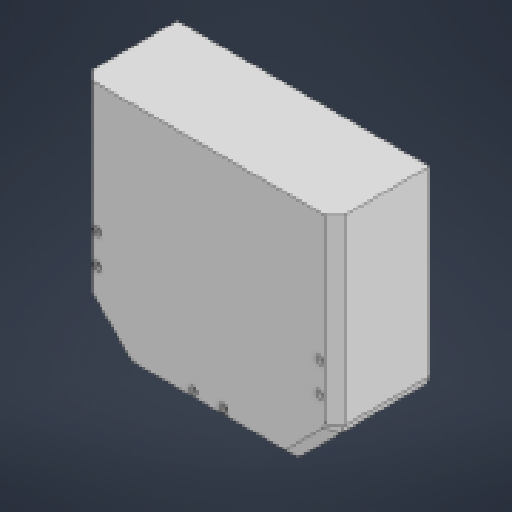
# Autodesk Inventor part: CNC-032-TopCover
Saved by Autodesk Inventor 2026.2 (Build 302298000, 298)
## iProperties
Created: 2026-06-28
Part Number: CNC-032-TopCover
Material: ABS Plastic
Document SubType Name: Modeling
Designer: Kenji
Density: 1.06 g/cm^3
Appearance: Smooth - White
Author: Kenji
Autodesk Inventor part; units mm, degrees
(part 1 of 2)
ref_plane "YZ Plane" through (0, 0, 0) normal (1, 0, 0) x (0, 1, 0)
ref_plane "XZ Plane" through (0, 0, 0) normal (0, 1, 0) x (-1, 0, 0)
ref_plane "XY Plane" through (0, 0, 0) normal (0, 0, 1) x (1, 0, 0)
ref_plane "Work Plane1" through (0, 0, 0) normal (0, 0, 1) x (1, 0, 0)
sketch "Sketch1" plane through (0, 0, 0) normal (0, 0, 1) x (1, 0, 0)
  arc A0 (66.7339, 54.005) -> (67.0931, 54.1538) centre (66.7339, 54.513) ccw construction
  line L0 (66.008, 54.005) -> (66.7339, 54.005) construction
  arc A1 (65.5, 54.513) -> (66.008, 54.005) centre (66.008, 54.513) ccw construction
  line L1 (65.5, 56.862) -> (65.5, 54.513) construction
  arc A2 (65.5, 56.862) -> (64.992, 57.37) centre (64.992, 56.862) ccw construction
  line L2 (64.508, 57.37) -> (64.992, 57.37) construction
  arc A3 (64.508, 57.37) -> (64, 56.862) centre (64.508, 56.862) ccw construction
  line L3 (64, 43.138) -> (64, 56.862) construction
  arc A4 (64, 43.138) -> (64.508, 42.63) centre (64.508, 43.138) ccw construction
  line L4 (64.992, 42.63) -> (64.508, 42.63) construction
  arc A5 (64.992, 42.63) -> (65.5, 43.138) centre (64.992, 43.138) ccw construction
  line L5 (65.5, 45.487) -> (65.5, 43.138) construction
  arc A6 (66.008, 45.995) -> (65.5, 45.487) centre (66.008, 45.487) ccw construction
  line L6 (66.7339, 45.995) -> (66.008, 45.995) construction
  arc A7 (67.0931, 45.8462) -> (66.7339, 45.995) centre (66.7339, 45.487) ccw construction
  line L7 (70.1962, 42.7431) -> (67.0931, 45.8462) construction
  arc A8 (70.345, 42.3839) -> (70.1962, 42.7431) centre (69.837, 42.3839) ccw construction
  line L8 (70.345, 37.6161) -> (70.345, 42.3839) construction
  arc A9 (70.1962, 37.2569) -> (70.345, 37.6161) centre (69.837, 37.6161) ccw construction
  line L9 (67.0931, 34.1538) -> (70.1962, 37.2569) construction
  arc A10 (66.7339, 34.005) -> (67.0931, 34.1538) centre (66.7339, 34.513) ccw construction
  line L10 (66.008, 34.005) -> (66.7339, 34.005) construction
  arc A11 (65.5, 34.513) -> (66.008, 34.005) centre (66.008, 34.513) ccw construction
  line L11 (65.5, 36.862) -> (65.5, 34.513) construction
  arc A12 (65.5, 36.862) -> (64.992, 37.37) centre (64.992, 36.862) ccw construction
  line L12 (64.508, 37.37) -> (64.992, 37.37) construction
  arc A13 (64.508, 37.37) -> (64, 36.862) centre (64.508, 36.862) ccw construction
  line L13 (64, 31.5) -> (64, 36.862) construction
  arc A14 (64, 31.5) -> (65.5, 30) centre (65.5, 31.5) ccw construction
  line L14 (70.862, 30) -> (65.5, 30) construction
  arc A15 (70.862, 30) -> (71.37, 30.508) centre (70.862, 30.508) ccw construction
  line L15 (71.37, 30.992) -> (71.37, 30.508) construction
  arc A16 (71.37, 30.992) -> (70.862, 31.5) centre (70.862, 30.992) ccw construction
  line L16 (68.513, 31.5) -> (70.862, 31.5) construction
  arc A17 (68.005, 32.008) -> (68.513, 31.5) centre (68.513, 32.008) ccw construction
  line L17 (68.005, 32.7339) -> (68.005, 32.008) construction
  arc A18 (68.1538, 33.0931) -> (68.005, 32.7339) centre (68.513, 32.7339) ccw construction
  line L18 (71.2569, 36.1962) -> (68.1538, 33.0931) construction
  arc A19 (71.6161, 36.345) -> (71.2569, 36.1962) centre (71.6161, 35.837) ccw construction
  line L19 (76.3839, 36.345) -> (71.6161, 36.345) construction
  arc A20 (76.7431, 36.1962) -> (76.3839, 36.345) centre (76.3839, 35.837) ccw construction
  line L20 (79.8462, 33.0931) -> (76.7431, 36.1962) construction
  arc A21 (79.995, 32.7339) -> (79.8462, 33.0931) centre (79.487, 32.7339) ccw construction
  line L21 (79.995, 32.008) -> (79.995, 32.7339) construction
  arc A22 (79.487, 31.5) -> (79.995, 32.008) centre (79.487, 32.008) ccw construction
  line L22 (77.138, 31.5) -> (79.487, 31.5) construction
  arc A23 (77.138, 31.5) -> (76.63, 30.992) centre (77.138, 30.992) ccw construction
  line L23 (76.63, 30.508) -> (76.63, 30.992) construction
  arc A24 (76.63, 30.508) -> (77.138, 30) centre (77.138, 30.508) ccw construction
  line L24 (82.5, 30) -> (77.138, 30) construction
  arc A25 (82.5, 30) -> (84, 31.5) centre (82.5, 31.5) ccw construction
  line L25 (84, 36.862) -> (84, 31.5) construction
  arc A26 (84, 36.862) -> (83.492, 37.37) centre (83.492, 36.862) ccw construction
  line L26 (83.008, 37.37) -> (83.492, 37.37) construction
  arc A27 (83.008, 37.37) -> (82.5, 36.862) centre (83.008, 36.862) ccw construction
  line L27 (82.5, 34.513) -> (82.5, 36.862) construction
  arc A28 (81.992, 34.005) -> (82.5, 34.513) centre (81.992, 34.513) ccw construction
  line L28 (81.2661, 34.005) -> (81.992, 34.005) construction
  arc A29 (80.9069, 34.1538) -> (81.2661, 34.005) centre (81.2661, 34.513) ccw construction
  line L29 (77.8038, 37.2569) -> (80.9069, 34.1538) construction
  arc A30 (77.655, 37.6161) -> (77.8038, 37.2569) centre (78.163, 37.6161) ccw construction
  line L30 (77.655, 42.3839) -> (77.655, 37.6161) construction
  arc A31 (77.8038, 42.7431) -> (77.655, 42.3839) centre (78.163, 42.3839) ccw construction
  line L31 (80.9069, 45.8462) -> (77.8038, 42.7431) construction
  arc A32 (81.2661, 45.995) -> (80.9069, 45.8462) centre (81.2661, 45.487) ccw construction
  line L32 (81.992, 45.995) -> (81.2661, 45.995) construction
  arc A33 (82.5, 45.487) -> (81.992, 45.995) centre (81.992, 45.487) ccw construction
  line L33 (82.5, 43.138) -> (82.5, 45.487) construction
  arc A34 (82.5, 43.138) -> (83.008, 42.63) centre (83.008, 43.138) ccw construction
  line L34 (83.492, 42.63) -> (83.008, 42.63) construction
  arc A35 (83.492, 42.63) -> (84, 43.138) centre (83.492, 43.138) ccw construction
  line L35 (84, 56.862) -> (84, 43.138) construction
  arc A36 (84, 56.862) -> (83.492, 57.37) centre (83.492, 56.862) ccw construction
  line L36 (83.008, 57.37) -> (83.492, 57.37) construction
  arc A37 (83.008, 57.37) -> (82.5, 56.862) centre (83.008, 56.862) ccw construction
  line L37 (82.5, 54.513) -> (82.5, 56.862) construction
  arc A38 (81.992, 54.005) -> (82.5, 54.513) centre (81.992, 54.513) ccw construction
  line L38 (81.2661, 54.005) -> (81.992, 54.005) construction
  arc A39 (80.9069, 54.1538) -> (81.2661, 54.005) centre (81.2661, 54.513) ccw construction
  line L39 (77.8038, 57.2569) -> (80.9069, 54.1538) construction
  arc A40 (77.655, 57.6161) -> (77.8038, 57.2569) centre (78.163, 57.6161) ccw construction
  line L40 (77.655, 62.3839) -> (77.655, 57.6161) construction
  arc A41 (77.8038, 62.7431) -> (77.655, 62.3839) centre (78.163, 62.3839) ccw construction
  line L41 (80.9069, 65.8462) -> (77.8038, 62.7431) construction
  arc A42 (81.2661, 65.995) -> (80.9069, 65.8462) centre (81.2661, 65.487) ccw construction
  line L42 (81.992, 65.995) -> (81.2661, 65.995) construction
  arc A43 (82.5, 65.487) -> (81.992, 65.995) centre (81.992, 65.487) ccw construction
  line L43 (82.5, 63.138) -> (82.5, 65.487) construction
  arc A44 (82.5, 63.138) -> (83.008, 62.63) centre (83.008, 63.138) ccw construction
  line L44 (83.492, 62.63) -> (83.008, 62.63) construction
  arc A45 (83.492, 62.63) -> (84, 63.138) centre (83.492, 63.138) ccw construction
  line L45 (84, 68.5) -> (84, 63.138) construction
  arc A46 (84, 68.5) -> (82.5, 70) centre (82.5, 68.5) ccw construction
  line L46 (77.138, 70) -> (82.5, 70) construction
  arc A47 (77.138, 70) -> (76.63, 69.492) centre (77.138, 69.492) ccw construction
  line L47 (76.63, 69.008) -> (76.63, 69.492) construction
  arc A48 (76.63, 69.008) -> (77.138, 68.5) centre (77.138, 69.008) ccw construction
  line L48 (79.487, 68.5) -> (77.138, 68.5) construction
  arc A49 (79.995, 67.992) -> (79.487, 68.5) centre (79.487, 67.992) ccw construction
  line L49 (79.995, 67.2661) -> (79.995, 67.992) construction
  arc A50 (79.8462, 66.9069) -> (79.995, 67.2661) centre (79.487, 67.2661) ccw construction
  line L50 (76.7431, 63.8038) -> (79.8462, 66.9069) construction
  arc A51 (76.3839, 63.655) -> (76.7431, 63.8038) centre (76.3839, 64.163) ccw construction
  line L51 (71.6161, 63.655) -> (76.3839, 63.655) construction
  arc A52 (71.2569, 63.8038) -> (71.6161, 63.655) centre (71.6161, 64.163) ccw construction
  line L52 (68.1538, 66.9069) -> (71.2569, 63.8038) construction
  arc A53 (68.005, 67.2661) -> (68.1538, 66.9069) centre (68.513, 67.2661) ccw construction
  line L53 (68.005, 67.992) -> (68.005, 67.2661) construction
  arc A54 (68.513, 68.5) -> (68.005, 67.992) centre (68.513, 67.992) ccw construction
  line L54 (70.862, 68.5) -> (68.513, 68.5) construction
  arc A55 (70.862, 68.5) -> (71.37, 69.008) centre (70.862, 69.008) ccw construction
  line L55 (71.37, 69.492) -> (71.37, 69.008) construction
  arc A56 (71.37, 69.492) -> (70.862, 70) centre (70.862, 69.492) ccw construction
  line L56 (65.5, 70) -> (70.862, 70) construction
  arc A57 (65.5, 70) -> (64, 68.5) centre (65.5, 68.5) ccw construction
  line L57 (64, 63.138) -> (64, 68.5) construction
  arc A58 (64, 63.138) -> (64.508, 62.63) centre (64.508, 63.138) ccw construction
  line L58 (64.992, 62.63) -> (64.508, 62.63) construction
  arc A59 (64.992, 62.63) -> (65.5, 63.138) centre (64.992, 63.138) ccw construction
  line L59 (65.5, 65.487) -> (65.5, 63.138) construction
  arc A60 (66.008, 65.995) -> (65.5, 65.487) centre (66.008, 65.487) ccw construction
  line L60 (66.7339, 65.995) -> (66.008, 65.995) construction
  arc A61 (67.0931, 65.8462) -> (66.7339, 65.995) centre (66.7339, 65.487) ccw construction
  line L61 (70.1962, 62.7431) -> (67.0931, 65.8462) construction
  arc A62 (70.345, 62.3839) -> (70.1962, 62.7431) centre (69.837, 62.3839) ccw construction
  line L62 (70.345, 57.6161) -> (70.345, 62.3839) construction
  arc A63 (70.1962, 57.2569) -> (70.345, 57.6161) centre (69.837, 57.6161) ccw construction
  line L63 (67.0931, 54.1538) -> (70.1962, 57.2569) construction
  arc A64 (71.6955, 42.1249) -> (72.0649, 40.804) centre (72.252, 41.5684) ccw construction
  line L64 (71.8751, 42.3045) -> (71.6955, 42.1249) construction
  arc A65 (73.196, 41.9351) -> (71.8751, 42.3045) centre (72.4316, 41.748) ccw construction
  arc A66 (74.804, 41.9351) -> (73.196, 41.9351) centre (74, 40) ccw construction
  arc A67 (76.1249, 42.3045) -> (74.804, 41.9351) centre (75.5684, 41.748) ccw construction
  line L65 (76.3045, 42.1249) -> (76.1249, 42.3045) construction
  arc A68 (75.9351, 40.804) -> (76.3045, 42.1249) centre (75.748, 41.5684) ccw construction
  arc A69 (75.9351, 39.196) -> (75.9351, 40.804) centre (74, 40) ccw construction
  arc A70 (76.3045, 37.8751) -> (75.9351, 39.196) centre (75.748, 38.4316) ccw construction
  line L66 (76.1249, 37.6955) -> (76.3045, 37.8751) construction
  arc A71 (74.804, 38.0649) -> (76.1249, 37.6955) centre (75.5684, 38.252) ccw construction
  arc A72 (73.196, 38.0649) -> (74.804, 38.0649) centre (74, 40) ccw construction
  arc A73 (71.8751, 37.6955) -> (73.196, 38.0649) centre (72.4316, 38.252) ccw construction
  line L67 (71.6955, 37.8751) -> (71.8751, 37.6955) construction
  arc A74 (72.0649, 39.196) -> (71.6955, 37.8751) centre (72.252, 38.4316) ccw construction
  arc A75 (72.0649, 40.804) -> (72.0649, 39.196) centre (74, 40) ccw construction
  arc A76 (67.3552, 52.505) -> (67.7144, 52.6538) centre (67.3552, 53.013) ccw construction
  line L68 (71.2569, 56.1962) -> (67.7144, 52.6538) construction
  arc A77 (71.6161, 56.345) -> (71.2569, 56.1962) centre (71.6161, 55.837) ccw construction
  line L69 (76.3839, 56.345) -> (71.6161, 56.345) construction
  arc A78 (76.7431, 56.1962) -> (76.3839, 56.345) centre (76.3839, 55.837) ccw construction
  line L70 (80.2856, 52.6538) -> (76.7431, 56.1962) construction
  arc A79 (80.2856, 52.6538) -> (80.6448, 52.505) centre (80.6448, 53.013) ccw construction
  line L71 (81.992, 52.505) -> (80.6448, 52.505) construction
  arc A80 (82.5, 51.997) -> (81.992, 52.505) centre (81.992, 51.997) ccw construction
  line L72 (82.5, 48.003) -> (82.5, 51.997) construction
  arc A81 (81.992, 47.495) -> (82.5, 48.003) centre (81.992, 48.003) ccw construction
  line L73 (80.6448, 47.495) -> (81.992, 47.495) construction
  arc A82 (80.6448, 47.495) -> (80.2856, 47.3462) centre (80.6448, 46.987) ccw construction
  line L74 (76.7431, 43.8038) -> (80.2856, 47.3462) construction
  arc A83 (76.3839, 43.655) -> (76.7431, 43.8038) centre (76.3839, 44.163) ccw construction
  line L75 (71.6161, 43.655) -> (76.3839, 43.655) construction
  arc A84 (71.2569, 43.8038) -> (71.6161, 43.655) centre (71.6161, 44.163) ccw construction
  line L76 (67.7144, 47.3462) -> (71.2569, 43.8038) construction
  arc A85 (67.7144, 47.3462) -> (67.3552, 47.495) centre (67.3552, 46.987) ccw construction
  line L77 (66.008, 47.495) -> (67.3552, 47.495) construction
  arc A86 (65.5, 48.003) -> (66.008, 47.495) centre (66.008, 48.003) ccw construction
  line L78 (65.5, 51.997) -> (65.5, 48.003) construction
  arc A87 (66.008, 52.505) -> (65.5, 51.997) centre (66.008, 51.997) ccw construction
  line L79 (67.3552, 52.505) -> (66.008, 52.505) construction
  arc A88 (71.6955, 62.1249) -> (72.0649, 60.804) centre (72.252, 61.5684) ccw construction
  line L80 (71.8751, 62.3045) -> (71.6955, 62.1249) construction
  arc A89 (73.196, 61.9351) -> (71.8751, 62.3045) centre (72.4316, 61.748) ccw construction
  arc A90 (74.804, 61.9351) -> (73.196, 61.9351) centre (74, 60) ccw construction
  arc A91 (76.1249, 62.3045) -> (74.804, 61.9351) centre (75.5684, 61.748) ccw construction
  line L81 (76.3045, 62.1249) -> (76.1249, 62.3045) construction
  arc A92 (75.9351, 60.804) -> (76.3045, 62.1249) centre (75.748, 61.5684) ccw construction
  arc A93 (75.9351, 59.196) -> (75.9351, 60.804) centre (74, 60) ccw construction
  arc A94 (76.3045, 57.8751) -> (75.9351, 59.196) centre (75.748, 58.4316) ccw construction
  line L82 (76.1249, 57.6955) -> (76.3045, 57.8751) construction
  arc A95 (74.804, 58.0649) -> (76.1249, 57.6955) centre (75.5684, 58.252) ccw construction
  arc A96 (73.196, 58.0649) -> (74.804, 58.0649) centre (74, 60) ccw construction
  arc A97 (71.8751, 57.6955) -> (73.196, 58.0649) centre (72.4316, 58.252) ccw construction
  line L83 (71.6955, 57.8751) -> (71.8751, 57.6955) construction
  arc A98 (72.0649, 59.196) -> (71.6955, 57.8751) centre (72.252, 58.4316) ccw construction
  arc A99 (72.0649, 60.804) -> (72.0649, 59.196) centre (74, 60) ccw construction
  arc A100 (-66.7339, 45.995) -> (-67.0931, 45.8462) centre (-66.7339, 45.487) ccw construction
  line L84 (-66.008, 45.995) -> (-66.7339, 45.995) construction
  arc A101 (-65.5, 45.487) -> (-66.008, 45.995) centre (-66.008, 45.487) ccw construction
  line L85 (-65.5, 43.138) -> (-65.5, 45.487) construction
  arc A102 (-65.5, 43.138) -> (-64.992, 42.63) centre (-64.992, 43.138) ccw construction
  line L86 (-64.508, 42.63) -> (-64.992, 42.63) construction
  arc A103 (-64.508, 42.63) -> (-64, 43.138) centre (-64.508, 43.138) ccw construction
  line L87 (-64, 56.862) -> (-64, 43.138) construction
  arc A104 (-64, 56.862) -> (-64.508, 57.37) centre (-64.508, 56.862) ccw construction
  line L88 (-64.992, 57.37) -> (-64.508, 57.37) construction
  arc A105 (-64.992, 57.37) -> (-65.5, 56.862) centre (-64.992, 56.862) ccw construction
  line L89 (-65.5, 54.513) -> (-65.5, 56.862) construction
  arc A106 (-66.008, 54.005) -> (-65.5, 54.513) centre (-66.008, 54.513) ccw construction
  line L90 (-66.7339, 54.005) -> (-66.008, 54.005) construction
  arc A107 (-67.0931, 54.1538) -> (-66.7339, 54.005) centre (-66.7339, 54.513) ccw construction
  line L91 (-70.1962, 57.2569) -> (-67.0931, 54.1538) construction
  arc A108 (-70.345, 57.6161) -> (-70.1962, 57.2569) centre (-69.837, 57.6161) ccw construction
  line L92 (-70.345, 62.3839) -> (-70.345, 57.6161) construction
  arc A109 (-70.1962, 62.7431) -> (-70.345, 62.3839) centre (-69.837, 62.3839) ccw construction
  line L93 (-67.0931, 65.8462) -> (-70.1962, 62.7431) construction
  arc A110 (-66.7339, 65.995) -> (-67.0931, 65.8462) centre (-66.7339, 65.487) ccw construction
  line L94 (-66.008, 65.995) -> (-66.7339, 65.995) construction
  arc A111 (-65.5, 65.487) -> (-66.008, 65.995) centre (-66.008, 65.487) ccw construction
  line L95 (-65.5, 63.138) -> (-65.5, 65.487) construction
  arc A112 (-65.5, 63.138) -> (-64.992, 62.63) centre (-64.992, 63.138) ccw construction
  line L96 (-64.508, 62.63) -> (-64.992, 62.63) construction
  arc A113 (-64.508, 62.63) -> (-64, 63.138) centre (-64.508, 63.138) ccw construction
  line L97 (-64, 68.5) -> (-64, 63.138) construction
  arc A114 (-64, 68.5) -> (-65.5, 70) centre (-65.5, 68.5) ccw construction
  line L98 (-70.862, 70) -> (-65.5, 70) construction
  arc A115 (-70.862, 70) -> (-71.37, 69.492) centre (-70.862, 69.492) ccw construction
  line L99 (-71.37, 69.008) -> (-71.37, 69.492) construction
  arc A116 (-71.37, 69.008) -> (-70.862, 68.5) centre (-70.862, 69.008) ccw construction
  line L100 (-68.513, 68.5) -> (-70.862, 68.5) construction
  arc A117 (-68.005, 67.992) -> (-68.513, 68.5) centre (-68.513, 67.992) ccw construction
  line L101 (-68.005, 67.2661) -> (-68.005, 67.992) construction
  arc A118 (-68.1538, 66.9069) -> (-68.005, 67.2661) centre (-68.513, 67.2661) ccw construction
  line L102 (-71.2569, 63.8038) -> (-68.1538, 66.9069) construction
  arc A119 (-71.6161, 63.655) -> (-71.2569, 63.8038) centre (-71.6161, 64.163) ccw construction
  line L103 (-76.3839, 63.655) -> (-71.6161, 63.655) construction
  arc A120 (-76.7431, 63.8038) -> (-76.3839, 63.655) centre (-76.3839, 64.163) ccw construction
  line L104 (-79.8462, 66.9069) -> (-76.7431, 63.8038) construction
  arc A121 (-79.995, 67.2661) -> (-79.8462, 66.9069) centre (-79.487, 67.2661) ccw construction
  line L105 (-79.995, 67.992) -> (-79.995, 67.2661) construction
  arc A122 (-79.487, 68.5) -> (-79.995, 67.992) centre (-79.487, 67.992) ccw construction
  line L106 (-77.138, 68.5) -> (-79.487, 68.5) construction
  arc A123 (-77.138, 68.5) -> (-76.63, 69.008) centre (-77.138, 69.008) ccw construction
  line L107 (-76.63, 69.492) -> (-76.63, 69.008) construction
  arc A124 (-76.63, 69.492) -> (-77.138, 70) centre (-77.138, 69.492) ccw construction
  line L108 (-82.5, 70) -> (-77.138, 70) construction
  arc A125 (-82.5, 70) -> (-84, 68.5) centre (-82.5, 68.5) ccw construction
  line L109 (-84, 63.138) -> (-84, 68.5) construction
  arc A126 (-84, 63.138) -> (-83.492, 62.63) centre (-83.492, 63.138) ccw construction
  line L110 (-83.008, 62.63) -> (-83.492, 62.63) construction
  arc A127 (-83.008, 62.63) -> (-82.5, 63.138) centre (-83.008, 63.138) ccw construction
  line L111 (-82.5, 65.487) -> (-82.5, 63.138) construction
  arc A128 (-81.992, 65.995) -> (-82.5, 65.487) centre (-81.992, 65.487) ccw construction
  line L112 (-81.2661, 65.995) -> (-81.992, 65.995) construction
  arc A129 (-80.9069, 65.8462) -> (-81.2661, 65.995) centre (-81.2661, 65.487) ccw construction
  line L113 (-77.8038, 62.7431) -> (-80.9069, 65.8462) construction
  arc A130 (-77.655, 62.3839) -> (-77.8038, 62.7431) centre (-78.163, 62.3839) ccw construction
  line L114 (-77.655, 57.6161) -> (-77.655, 62.3839) construction
  arc A131 (-77.8038, 57.2569) -> (-77.655, 57.6161) centre (-78.163, 57.6161) ccw construction
  line L115 (-80.9069, 54.1538) -> (-77.8038, 57.2569) construction
  arc A132 (-81.2661, 54.005) -> (-80.9069, 54.1538) centre (-81.2661, 54.513) ccw construction
  line L116 (-81.992, 54.005) -> (-81.2661, 54.005) construction
  arc A133 (-82.5, 54.513) -> (-81.992, 54.005) centre (-81.992, 54.513) ccw construction
  line L117 (-82.5, 56.862) -> (-82.5, 54.513) construction
  arc A134 (-82.5, 56.862) -> (-83.008, 57.37) centre (-83.008, 56.862) ccw construction
  line L118 (-83.492, 57.37) -> (-83.008, 57.37) construction
  arc A135 (-83.492, 57.37) -> (-84, 56.862) centre (-83.492, 56.862) ccw construction
  line L119 (-84, 43.138) -> (-84, 56.862) construction
  arc A136 (-84, 43.138) -> (-83.492, 42.63) centre (-83.492, 43.138) ccw construction
  line L120 (-83.008, 42.63) -> (-83.492, 42.63) construction
  arc A137 (-83.008, 42.63) -> (-82.5, 43.138) centre (-83.008, 43.138) ccw construction
  line L121 (-82.5, 45.487) -> (-82.5, 43.138) construction
  arc A138 (-81.992, 45.995) -> (-82.5, 45.487) centre (-81.992, 45.487) ccw construction
  line L122 (-81.2661, 45.995) -> (-81.992, 45.995) construction
  arc A139 (-80.9069, 45.8462) -> (-81.2661, 45.995) centre (-81.2661, 45.487) ccw construction
  line L123 (-77.8038, 42.7431) -> (-80.9069, 45.8462) construction
  arc A140 (-77.655, 42.3839) -> (-77.8038, 42.7431) centre (-78.163, 42.3839) ccw construction
  line L124 (-77.655, 37.6161) -> (-77.655, 42.3839) construction
  arc A141 (-77.8038, 37.2569) -> (-77.655, 37.6161) centre (-78.163, 37.6161) ccw construction
  line L125 (-80.9069, 34.1538) -> (-77.8038, 37.2569) construction
  arc A142 (-81.2661, 34.005) -> (-80.9069, 34.1538) centre (-81.2661, 34.513) ccw construction
  line L126 (-81.992, 34.005) -> (-81.2661, 34.005) construction
  arc A143 (-82.5, 34.513) -> (-81.992, 34.005) centre (-81.992, 34.513) ccw construction
  line L127 (-82.5, 36.862) -> (-82.5, 34.513) construction
  arc A144 (-82.5, 36.862) -> (-83.008, 37.37) centre (-83.008, 36.862) ccw construction
  line L128 (-83.492, 37.37) -> (-83.008, 37.37) construction
  arc A145 (-83.492, 37.37) -> (-84, 36.862) centre (-83.492, 36.862) ccw construction
  line L129 (-84, 31.5) -> (-84, 36.862) construction
  arc A146 (-84, 31.5) -> (-82.5, 30) centre (-82.5, 31.5) ccw construction
  line L130 (-77.138, 30) -> (-82.5, 30) construction
  arc A147 (-77.138, 30) -> (-76.63, 30.508) centre (-77.138, 30.508) ccw construction
  line L131 (-76.63, 30.992) -> (-76.63, 30.508) construction
  arc A148 (-76.63, 30.992) -> (-77.138, 31.5) centre (-77.138, 30.992) ccw construction
  line L132 (-79.487, 31.5) -> (-77.138, 31.5) construction
  arc A149 (-79.995, 32.008) -> (-79.487, 31.5) centre (-79.487, 32.008) ccw construction
  line L133 (-79.995, 32.7339) -> (-79.995, 32.008) construction
  arc A150 (-79.8462, 33.0931) -> (-79.995, 32.7339) centre (-79.487, 32.7339) ccw construction
  line L134 (-76.7431, 36.1962) -> (-79.8462, 33.0931) construction
  arc A151 (-76.3839, 36.345) -> (-76.7431, 36.1962) centre (-76.3839, 35.837) ccw construction
  line L135 (-71.6161, 36.345) -> (-76.3839, 36.345) construction
  arc A152 (-71.2569, 36.1962) -> (-71.6161, 36.345) centre (-71.6161, 35.837) ccw construction
  line L136 (-68.1538, 33.0931) -> (-71.2569, 36.1962) construction
  arc A153 (-68.005, 32.7339) -> (-68.1538, 33.0931) centre (-68.513, 32.7339) ccw construction
  line L137 (-68.005, 32.008) -> (-68.005, 32.7339) construction
  arc A154 (-68.513, 31.5) -> (-68.005, 32.008) centre (-68.513, 32.008) ccw construction
  line L138 (-70.862, 31.5) -> (-68.513, 31.5) construction
  arc A155 (-70.862, 31.5) -> (-71.37, 30.992) centre (-70.862, 30.992) ccw construction
  line L139 (-71.37, 30.508) -> (-71.37, 30.992) construction
  arc A156 (-71.37, 30.508) -> (-70.862, 30) centre (-70.862, 30.508) ccw construction
  line L140 (-65.5, 30) -> (-70.862, 30) construction
  arc A157 (-65.5, 30) -> (-64, 31.5) centre (-65.5, 31.5) ccw construction
  line L141 (-64, 36.862) -> (-64, 31.5) construction
  arc A158 (-64, 36.862) -> (-64.508, 37.37) centre (-64.508, 36.862) ccw construction
  line L142 (-64.992, 37.37) -> (-64.508, 37.37) construction
  arc A159 (-64.992, 37.37) -> (-65.5, 36.862) centre (-64.992, 36.862) ccw construction
  line L143 (-65.5, 34.513) -> (-65.5, 36.862) construction
  arc A160 (-66.008, 34.005) -> (-65.5, 34.513) centre (-66.008, 34.513) ccw construction
  line L144 (-66.7339, 34.005) -> (-66.008, 34.005) construction
  arc A161 (-67.0931, 34.1538) -> (-66.7339, 34.005) centre (-66.7339, 34.513) ccw construction
  line L145 (-70.1962, 37.2569) -> (-67.0931, 34.1538) construction
  arc A162 (-70.345, 37.6161) -> (-70.1962, 37.2569) centre (-69.837, 37.6161) ccw construction
  line L146 (-70.345, 42.3839) -> (-70.345, 37.6161) construction
  arc A163 (-70.1962, 42.7431) -> (-70.345, 42.3839) centre (-69.837, 42.3839) ccw construction
  line L147 (-67.0931, 45.8462) -> (-70.1962, 42.7431) construction
  arc A164 (-71.6955, 57.8751) -> (-72.0649, 59.196) centre (-72.252, 58.4316) ccw construction
  line L148 (-71.8751, 57.6955) -> (-71.6955, 57.8751) construction
  arc A165 (-73.196, 58.0649) -> (-71.8751, 57.6955) centre (-72.4316, 58.252) ccw construction
  arc A166 (-74.804, 58.0649) -> (-73.196, 58.0649) centre (-74, 60) ccw construction
  arc A167 (-76.1249, 57.6955) -> (-74.804, 58.0649) centre (-75.5684, 58.252) ccw construction
  line L149 (-76.3045, 57.8751) -> (-76.1249, 57.6955) construction
  arc A168 (-75.9351, 59.196) -> (-76.3045, 57.8751) centre (-75.748, 58.4316) ccw construction
  arc A169 (-75.9351, 60.804) -> (-75.9351, 59.196) centre (-74, 60) ccw construction
  arc A170 (-76.3045, 62.1249) -> (-75.9351, 60.804) centre (-75.748, 61.5684) ccw construction
  line L150 (-76.1249, 62.3045) -> (-76.3045, 62.1249) construction
  arc A171 (-74.804, 61.9351) -> (-76.1249, 62.3045) centre (-75.5684, 61.748) ccw construction
  arc A172 (-73.196, 61.9351) -> (-74.804, 61.9351) centre (-74, 60) ccw construction
  arc A173 (-71.8751, 62.3045) -> (-73.196, 61.9351) centre (-72.4316, 61.748) ccw construction
  line L151 (-71.6955, 62.1249) -> (-71.8751, 62.3045) construction
  arc A174 (-72.0649, 60.804) -> (-71.6955, 62.1249) centre (-72.252, 61.5684) ccw construction
  arc A175 (-72.0649, 59.196) -> (-72.0649, 60.804) centre (-74, 60) ccw construction
  arc A176 (-67.3552, 47.495) -> (-67.7144, 47.3462) centre (-67.3552, 46.987) ccw construction
  line L152 (-71.2569, 43.8038) -> (-67.7144, 47.3462) construction
  arc A177 (-71.6161, 43.655) -> (-71.2569, 43.8038) centre (-71.6161, 44.163) ccw construction
  line L153 (-76.3839, 43.655) -> (-71.6161, 43.655) construction
  arc A178 (-76.7431, 43.8038) -> (-76.3839, 43.655) centre (-76.3839, 44.163) ccw construction
  line L154 (-80.2856, 47.3462) -> (-76.7431, 43.8038) construction
  arc A179 (-80.2856, 47.3462) -> (-80.6448, 47.495) centre (-80.6448, 46.987) ccw construction
  line L155 (-81.992, 47.495) -> (-80.6448, 47.495) construction
  arc A180 (-82.5, 48.003) -> (-81.992, 47.495) centre (-81.992, 48.003) ccw construction
  line L156 (-82.5, 51.997) -> (-82.5, 48.003) construction
  arc A181 (-81.992, 52.505) -> (-82.5, 51.997) centre (-81.992, 51.997) ccw construction
  line L157 (-80.6448, 52.505) -> (-81.992, 52.505) construction
  arc A182 (-80.6448, 52.505) -> (-80.2856, 52.6538) centre (-80.6448, 53.013) ccw construction
  line L158 (-76.7431, 56.1962) -> (-80.2856, 52.6538) construction
  arc A183 (-76.3839, 56.345) -> (-76.7431, 56.1962) centre (-76.3839, 55.837) ccw construction
  line L159 (-71.6161, 56.345) -> (-76.3839, 56.345) construction
  arc A184 (-71.2569, 56.1962) -> (-71.6161, 56.345) centre (-71.6161, 55.837) ccw construction
  line L160 (-67.7144, 52.6538) -> (-71.2569, 56.1962) construction
  arc A185 (-67.7144, 52.6538) -> (-67.3552, 52.505) centre (-67.3552, 53.013) ccw construction
  line L161 (-66.008, 52.505) -> (-67.3552, 52.505) construction
  arc A186 (-65.5, 51.997) -> (-66.008, 52.505) centre (-66.008, 51.997) ccw construction
  line L162 (-65.5, 48.003) -> (-65.5, 51.997) construction
  arc A187 (-66.008, 47.495) -> (-65.5, 48.003) centre (-66.008, 48.003) ccw construction
  line L163 (-67.3552, 47.495) -> (-66.008, 47.495) construction
  arc A188 (-71.6955, 37.8751) -> (-72.0649, 39.196) centre (-72.252, 38.4316) ccw construction
  line L164 (-71.8751, 37.6955) -> (-71.6955, 37.8751) construction
  arc A189 (-73.196, 38.0649) -> (-71.8751, 37.6955) centre (-72.4316, 38.252) ccw construction
  arc A190 (-74.804, 38.0649) -> (-73.196, 38.0649) centre (-74, 40) ccw construction
  arc A191 (-76.1249, 37.6955) -> (-74.804, 38.0649) centre (-75.5684, 38.252) ccw construction
  line L165 (-76.3045, 37.8751) -> (-76.1249, 37.6955) construction
  arc A192 (-75.9351, 39.196) -> (-76.3045, 37.8751) centre (-75.748, 38.4316) ccw construction
  arc A193 (-75.9351, 40.804) -> (-75.9351, 39.196) centre (-74, 40) ccw construction
  arc A194 (-76.3045, 42.1249) -> (-75.9351, 40.804) centre (-75.748, 41.5684) ccw construction
  line L166 (-76.1249, 42.3045) -> (-76.3045, 42.1249) construction
  arc A195 (-74.804, 41.9351) -> (-76.1249, 42.3045) centre (-75.5684, 41.748) ccw construction
  arc A196 (-73.196, 41.9351) -> (-74.804, 41.9351) centre (-74, 40) ccw construction
  arc A197 (-71.8751, 42.3045) -> (-73.196, 41.9351) centre (-72.4316, 41.748) ccw construction
  line L167 (-71.6955, 42.1249) -> (-71.8751, 42.3045) construction
  arc A198 (-72.0649, 40.804) -> (-71.6955, 42.1249) centre (-72.252, 41.5684) ccw construction
  arc A199 (-72.0649, 39.196) -> (-72.0649, 40.804) centre (-74, 40) ccw construction
  line L168 (13.138, -10) -> (18.5, -10) construction
  arc A200 (18.5, -10) -> (20, -8.5) centre (18.5, -8.5) ccw construction
  line L169 (20, -8.5) -> (20, -3.138) construction
  arc A201 (20, -3.138) -> (19.492, -2.63) centre (19.492, -3.138) ccw construction
  line L170 (19.492, -2.63) -> (19.008, -2.63) construction
  arc A202 (19.008, -2.63) -> (18.5, -3.138) centre (19.008, -3.138) ccw construction
  line L171 (18.5, -3.138) -> (18.5, -5.487) construction
  arc A203 (17.992, -5.995) -> (18.5, -5.487) centre (17.992, -5.487) ccw construction
  line L172 (17.992, -5.995) -> (17.2661, -5.995) construction
  arc A204 (16.9069, -5.8462) -> (17.2661, -5.995) centre (17.2661, -5.487) ccw construction
  line L173 (16.9069, -5.8462) -> (13.8038, -2.7431) construction
  arc A205 (13.655, -2.3839) -> (13.8038, -2.7431) centre (14.163, -2.3839) ccw construction
  line L174 (13.655, -2.3839) -> (13.655, 2.3839) construction
  arc A206 (13.8038, 2.7431) -> (13.655, 2.3839) centre (14.163, 2.3839) ccw construction
  line L175 (13.8038, 2.7431) -> (16.9069, 5.8462) construction
  arc A207 (17.2661, 5.995) -> (16.9069, 5.8462) centre (17.2661, 5.487) ccw construction
  line L176 (17.2661, 5.995) -> (17.992, 5.995) construction
  arc A208 (18.5, 5.487) -> (17.992, 5.995) centre (17.992, 5.487) ccw construction
  line L177 (18.5, 5.487) -> (18.5, 3.138) construction
  arc A209 (18.5, 3.138) -> (19.008, 2.63) centre (19.008, 3.138) ccw construction
  line L178 (19.008, 2.63) -> (19.492, 2.63) construction
  arc A210 (19.492, 2.63) -> (20, 3.138) centre (19.492, 3.138) ccw construction
  line L179 (20, 3.138) -> (20, 8.5) construction
  arc A211 (20, 8.5) -> (18.5, 10) centre (18.5, 8.5) ccw construction
  line L180 (18.5, 10) -> (13.138, 10) construction
  arc A212 (13.138, 10) -> (12.63, 9.492) centre (13.138, 9.492) ccw construction
  line L181 (12.63, 9.492) -> (12.63, 9.008) construction
  arc A213 (12.63, 9.008) -> (13.138, 8.5) centre (13.138, 9.008) ccw construction
  line L182 (13.138, 8.5) -> (15.487, 8.5) construction
  arc A214 (15.995, 7.992) -> (15.487, 8.5) centre (15.487, 7.992) ccw construction
  line L183 (15.995, 7.992) -> (15.995, 7.2661) construction
  arc A215 (15.8462, 6.9069) -> (15.995, 7.2661) centre (15.487, 7.2661) ccw construction
  line L184 (15.8462, 6.9069) -> (12.7431, 3.8038) construction
  arc A216 (12.3839, 3.655) -> (12.7431, 3.8038) centre (12.3839, 4.163) ccw construction
  line L185 (12.3839, 3.655) -> (7.6161, 3.655) construction
  arc A217 (7.2569, 3.8038) -> (7.6161, 3.655) centre (7.6161, 4.163) ccw construction
  line L186 (7.2569, 3.8038) -> (4.1538, 6.9069) construction
  arc A218 (4.005, 7.2661) -> (4.1538, 6.9069) centre (4.513, 7.2661) ccw construction
  line L187 (4.005, 7.2661) -> (4.005, 7.992) construction
  arc A219 (4.513, 8.5) -> (4.005, 7.992) centre (4.513, 7.992) ccw construction
  line L188 (4.513, 8.5) -> (6.862, 8.5) construction
  arc A220 (6.862, 8.5) -> (7.37, 9.008) centre (6.862, 9.008) ccw construction
  line L189 (7.37, 9.008) -> (7.37, 9.492) construction
  arc A221 (7.37, 9.492) -> (6.862, 10) centre (6.862, 9.492) ccw construction
  line L190 (6.862, 10) -> (-6.862, 10) construction
  arc A222 (-6.862, 10) -> (-7.37, 9.492) centre (-6.862, 9.492) ccw construction
  line L191 (-7.37, 9.492) -> (-7.37, 9.008) construction
  arc A223 (-7.37, 9.008) -> (-6.862, 8.5) centre (-6.862, 9.008) ccw construction
  line L192 (-6.862, 8.5) -> (-4.513, 8.5) construction
  arc A224 (-4.005, 7.992) -> (-4.513, 8.5) centre (-4.513, 7.992) ccw construction
  line L193 (-4.005, 7.992) -> (-4.005, 7.2661) construction
  arc A225 (-4.1538, 6.9069) -> (-4.005, 7.2661) centre (-4.513, 7.2661) ccw construction
  line L194 (-4.1538, 6.9069) -> (-7.2569, 3.8038) construction
  arc A226 (-7.6161, 3.655) -> (-7.2569, 3.8038) centre (-7.6161, 4.163) ccw construction
  line L195 (-7.6161, 3.655) -> (-12.3839, 3.655) construction
  arc A227 (-12.7431, 3.8038) -> (-12.3839, 3.655) centre (-12.3839, 4.163) ccw construction
  line L196 (-12.7431, 3.8038) -> (-15.8462, 6.9069) construction
  arc A228 (-15.995, 7.2661) -> (-15.8462, 6.9069) centre (-15.487, 7.2661) ccw construction
  line L197 (-15.995, 7.2661) -> (-15.995, 7.992) construction
  arc A229 (-15.487, 8.5) -> (-15.995, 7.992) centre (-15.487, 7.992) ccw construction
  line L198 (-15.487, 8.5) -> (-13.138, 8.5) construction
  arc A230 (-13.138, 8.5) -> (-12.63, 9.008) centre (-13.138, 9.008) ccw construction
  line L199 (-12.63, 9.008) -> (-12.63, 9.492) construction
  arc A231 (-12.63, 9.492) -> (-13.138, 10) centre (-13.138, 9.492) ccw construction
  line L200 (-13.138, 10) -> (-18.5, 10) construction
  arc A232 (-18.5, 10) -> (-20, 8.5) centre (-18.5, 8.5) ccw construction
  line L201 (-20, 8.5) -> (-20, 3.138) construction
  arc A233 (-20, 3.138) -> (-19.492, 2.63) centre (-19.492, 3.138) ccw construction
  line L202 (-19.492, 2.63) -> (-19.008, 2.63) construction
  arc A234 (-19.008, 2.63) -> (-18.5, 3.138) centre (-19.008, 3.138) ccw construction
  line L203 (-18.5, 3.138) -> (-18.5, 5.487) construction
  arc A235 (-17.992, 5.995) -> (-18.5, 5.487) centre (-17.992, 5.487) ccw construction
  line L204 (-17.992, 5.995) -> (-17.2661, 5.995) construction
  arc A236 (-16.9069, 5.8462) -> (-17.2661, 5.995) centre (-17.2661, 5.487) ccw construction
  line L205 (-16.9069, 5.8462) -> (-13.8038, 2.7431) construction
  arc A237 (-13.655, 2.3839) -> (-13.8038, 2.7431) centre (-14.163, 2.3839) ccw construction
  line L206 (-13.655, 2.3839) -> (-13.655, -2.3839) construction
  arc A238 (-13.8038, -2.7431) -> (-13.655, -2.3839) centre (-14.163, -2.3839) ccw construction
  line L207 (-13.8038, -2.7431) -> (-16.9069, -5.8462) construction
  arc A239 (-17.2661, -5.995) -> (-16.9069, -5.8462) centre (-17.2661, -5.487) ccw construction
  line L208 (-17.2661, -5.995) -> (-17.992, -5.995) construction
  arc A240 (-18.5, -5.487) -> (-17.992, -5.995) centre (-17.992, -5.487) ccw construction
  line L209 (-18.5, -5.487) -> (-18.5, -3.138) construction
  arc A241 (-18.5, -3.138) -> (-19.008, -2.63) centre (-19.008, -3.138) ccw construction
  line L210 (-19.008, -2.63) -> (-19.492, -2.63) construction
  arc A242 (-19.492, -2.63) -> (-20, -3.138) centre (-19.492, -3.138) ccw construction
  line L211 (-20, -3.138) -> (-20, -8.5) construction
  arc A243 (-20, -8.5) -> (-18.5, -10) centre (-18.5, -8.5) ccw construction
  line L212 (-18.5, -10) -> (-13.138, -10) construction
  arc A244 (-13.138, -10) -> (-12.63, -9.492) centre (-13.138, -9.492) ccw construction
  line L213 (-12.63, -9.492) -> (-12.63, -9.008) construction
  arc A245 (-12.63, -9.008) -> (-13.138, -8.5) centre (-13.138, -9.008) ccw construction
  line L214 (-13.138, -8.5) -> (-15.487, -8.5) construction
  arc A246 (-15.995, -7.992) -> (-15.487, -8.5) centre (-15.487, -7.992) ccw construction
  line L215 (-15.995, -7.992) -> (-15.995, -7.2661) construction
  arc A247 (-15.8462, -6.9069) -> (-15.995, -7.2661) centre (-15.487, -7.2661) ccw construction
  line L216 (-15.8462, -6.9069) -> (-12.7431, -3.8038) construction
  arc A248 (-12.3839, -3.655) -> (-12.7431, -3.8038) centre (-12.3839, -4.163) ccw construction
  line L217 (-12.3839, -3.655) -> (-7.6161, -3.655) construction
  arc A249 (-7.2569, -3.8038) -> (-7.6161, -3.655) centre (-7.6161, -4.163) ccw construction
  line L218 (-7.2569, -3.8038) -> (-4.1538, -6.9069) construction
  arc A250 (-4.005, -7.2661) -> (-4.1538, -6.9069) centre (-4.513, -7.2661) ccw construction
  line L219 (-4.005, -7.2661) -> (-4.005, -7.992) construction
  arc A251 (-4.513, -8.5) -> (-4.005, -7.992) centre (-4.513, -7.992) ccw construction
  line L220 (-4.513, -8.5) -> (-6.862, -8.5) construction
  arc A252 (-6.862, -8.5) -> (-7.37, -9.008) centre (-6.862, -9.008) ccw construction
  line L221 (-7.37, -9.008) -> (-7.37, -9.492) construction
  arc A253 (-7.37, -9.492) -> (-6.862, -10) centre (-6.862, -9.492) ccw construction
  line L222 (-6.862, -10) -> (6.862, -10) construction
  arc A254 (6.862, -10) -> (7.37, -9.492) centre (6.862, -9.492) ccw construction
  line L223 (7.37, -9.492) -> (7.37, -9.008) construction
  arc A255 (7.37, -9.008) -> (6.862, -8.5) centre (6.862, -9.008) ccw construction
  line L224 (6.862, -8.5) -> (4.513, -8.5) construction
  arc A256 (4.005, -7.992) -> (4.513, -8.5) centre (4.513, -7.992) ccw construction
  line L225 (4.005, -7.992) -> (4.005, -7.2661) construction
  arc A257 (4.1538, -6.9069) -> (4.005, -7.2661) centre (4.513, -7.2661) ccw construction
  line L226 (4.1538, -6.9069) -> (7.2569, -3.8038) construction
  arc A258 (7.6161, -3.655) -> (7.2569, -3.8038) centre (7.6161, -4.163) ccw construction
  line L227 (7.6161, -3.655) -> (12.3839, -3.655) construction
  arc A259 (12.7431, -3.8038) -> (12.3839, -3.655) centre (12.3839, -4.163) ccw construction
  line L228 (12.7431, -3.8038) -> (15.8462, -6.9069) construction
  arc A260 (15.995, -7.2661) -> (15.8462, -6.9069) centre (15.487, -7.2661) ccw construction
  line L229 (15.995, -7.2661) -> (15.995, -7.992) construction
  arc A261 (15.487, -8.5) -> (15.995, -7.992) centre (15.487, -7.992) ccw construction
  line L230 (15.487, -8.5) -> (13.138, -8.5) construction
  arc A262 (13.138, -8.5) -> (12.63, -9.008) centre (13.138, -9.008) ccw construction
  line L231 (12.63, -9.008) -> (12.63, -9.492) construction
  arc A263 (12.63, -9.492) -> (13.138, -10) centre (13.138, -9.492) ccw construction
  line L232 (12.3045, -2.1249) -> (12.1249, -2.3045) construction
  arc A264 (10.804, -1.9351) -> (12.1249, -2.3045) centre (11.5684, -1.748) ccw construction
  arc A265 (9.196, -1.9351) -> (10.804, -1.9351) centre (10, 0) ccw construction
  arc A266 (7.8751, -2.3045) -> (9.196, -1.9351) centre (8.4316, -1.748) ccw construction
  line L233 (7.8751, -2.3045) -> (7.6955, -2.1249) construction
  arc A267 (8.0649, -0.804) -> (7.6955, -2.1249) centre (8.252, -1.5684) ccw construction
  arc A268 (8.0649, 0.804) -> (8.0649, -0.804) centre (10, 0) ccw construction
  arc A269 (7.6955, 2.1249) -> (8.0649, 0.804) centre (8.252, 1.5684) ccw construction
  line L234 (7.6955, 2.1249) -> (7.8751, 2.3045) construction
  arc A270 (9.196, 1.9351) -> (7.8751, 2.3045) centre (8.4316, 1.748) ccw construction
  arc A271 (10.804, 1.9351) -> (9.196, 1.9351) centre (10, 0) ccw construction
  arc A272 (12.1249, 2.3045) -> (10.804, 1.9351) centre (11.5684, 1.748) ccw construction
  line L235 (12.1249, 2.3045) -> (12.3045, 2.1249) construction
  arc A273 (11.9351, 0.804) -> (12.3045, 2.1249) centre (11.748, 1.5684) ccw construction
  arc A274 (11.9351, -0.804) -> (11.9351, 0.804) centre (10, 0) ccw construction
  arc A275 (12.3045, -2.1249) -> (11.9351, -0.804) centre (11.748, -1.5684) ccw construction
  line L236 (-12.3045, 2.1249) -> (-12.1249, 2.3045) construction
  arc A276 (-10.804, 1.9351) -> (-12.1249, 2.3045) centre (-11.5684, 1.748) ccw construction
  arc A277 (-9.196, 1.9351) -> (-10.804, 1.9351) centre (-10, 0) ccw construction
  arc A278 (-7.8751, 2.3045) -> (-9.196, 1.9351) centre (-8.4316, 1.748) ccw construction
  line L237 (-7.8751, 2.3045) -> (-7.6955, 2.1249) construction
  arc A279 (-8.0649, 0.804) -> (-7.6955, 2.1249) centre (-8.252, 1.5684) ccw construction
  arc A280 (-8.0649, -0.804) -> (-8.0649, 0.804) centre (-10, 0) ccw construction
  arc A281 (-7.6955, -2.1249) -> (-8.0649, -0.804) centre (-8.252, -1.5684) ccw construction
  line L238 (-7.6955, -2.1249) -> (-7.8751, -2.3045) construction
  arc A282 (-9.196, -1.9351) -> (-7.8751, -2.3045) centre (-8.4316, -1.748) ccw construction
  arc A283 (-10.804, -1.9351) -> (-9.196, -1.9351) centre (-10, 0) ccw construction
  arc A284 (-12.1249, -2.3045) -> (-10.804, -1.9351) centre (-11.5684, -1.748) ccw construction
  line L239 (-12.1249, -2.3045) -> (-12.3045, -2.1249) construction
  arc A285 (-11.9351, -0.804) -> (-12.3045, -2.1249) centre (-11.748, -1.5684) ccw construction
  arc A286 (-11.9351, 0.804) -> (-11.9351, -0.804) centre (-10, 0) ccw construction
  arc A287 (-12.3045, 2.1249) -> (-11.9351, 0.804) centre (-11.748, 1.5684) ccw construction
  arc A288 (2.505, 6.6448) -> (2.6538, 6.2856) centre (3.013, 6.6448) ccw construction
  line L240 (2.6538, 6.2856) -> (6.1962, 2.7431) construction
  arc A289 (6.345, 2.3839) -> (6.1962, 2.7431) centre (5.837, 2.3839) ccw construction
  line L241 (6.345, 2.3839) -> (6.345, -2.3839) construction
  arc A290 (6.1962, -2.7431) -> (6.345, -2.3839) centre (5.837, -2.3839) ccw construction
  line L242 (6.1962, -2.7431) -> (2.6538, -6.2856) construction
  arc A291 (2.6538, -6.2856) -> (2.505, -6.6448) centre (3.013, -6.6448) ccw construction
  line L243 (2.505, -6.6448) -> (2.505, -7.992) construction
  arc A292 (1.997, -8.5) -> (2.505, -7.992) centre (1.997, -7.992) ccw construction
  line L244 (1.997, -8.5) -> (-1.997, -8.5) construction
  arc A293 (-2.505, -7.992) -> (-1.997, -8.5) centre (-1.997, -7.992) ccw construction
  line L245 (-2.505, -7.992) -> (-2.505, -6.6448) construction
  arc A294 (-2.505, -6.6448) -> (-2.6538, -6.2856) centre (-3.013, -6.6448) ccw construction
  line L246 (-2.6538, -6.2856) -> (-6.1962, -2.7431) construction
  arc A295 (-6.345, -2.3839) -> (-6.1962, -2.7431) centre (-5.837, -2.3839) ccw construction
  line L247 (-6.345, -2.3839) -> (-6.345, 2.3839) construction
  arc A296 (-6.1962, 2.7431) -> (-6.345, 2.3839) centre (-5.837, 2.3839) ccw construction
  line L248 (-6.1962, 2.7431) -> (-2.6538, 6.2856) construction
  arc A297 (-2.6538, 6.2856) -> (-2.505, 6.6448) centre (-3.013, 6.6448) ccw construction
  line L249 (-2.505, 6.6448) -> (-2.505, 7.992) construction
  arc A298 (-1.997, 8.5) -> (-2.505, 7.992) centre (-1.997, 7.992) ccw construction
  line L250 (-1.997, 8.5) -> (1.997, 8.5) construction
  arc A299 (2.505, 7.992) -> (1.997, 8.5) centre (1.997, 7.992) ccw construction
  line L251 (2.505, 7.992) -> (2.505, 6.6448) construction
  line L252 (78, 145) -> (-78, 145) construction
  line L253 (0, -10) -> (50.35, -10)
  line L254 (20, 30) -> (84, 30) construction
  line L255 (20, -10) -> (20, 30) construction
  line L256 (50.35, -10) -> (20, -10) projected
  line L257 (50.35, -10) -> (55.7701, -7.7549) projected
  line L258 (81.7549, 18.2299) -> (55.7701, -7.7549) projected
  line L259 (81.7549, 18.2299) -> (84, 23.65) projected
  line L260 (84, 30) -> (84, 23.65) projected
  line L261 (79.2375, 25.2375) -> (40, 25.2375) construction
  line L262 (79.2375, 22.4477) -> (79.2375, 25.2375) construction
  line L263 (51.5523, -5.2375) -> (79.2375, 22.4477) construction
  line L264 (24.7625, -5.2375) -> (51.5523, -5.2375) construction
  line L265 (24.7625, 10) -> (24.7625, -5.2375) construction
  line L266 (40, 25.2375) -> (24.7625, 10) construction
  line L267 (-20, 30) -> (-84, 30) construction
  line L268 (-84, 30) -> (-84, 23.65) projected
  line L269 (-81.7549, 18.2299) -> (-84, 23.65) projected
  line L270 (-81.7549, 18.2299) -> (-55.7701, -7.7549) projected
  line L271 (-50.35, -10) -> (-55.7701, -7.7549) projected
  line L272 (-50.35, -10) -> (-20, -10) projected
  line L273 (-20, -10) -> (-20, 30) construction
  line L274 (-79.2375, 25.2375) -> (-40, 25.2375) construction
  line L275 (-40, 25.2375) -> (-24.7625, 10) construction
  line L276 (-24.7625, 10) -> (-24.7625, -5.2375) construction
  line L277 (-24.7625, -5.2375) -> (-51.5523, -5.2375) construction
  line L278 (-51.5523, -5.2375) -> (-79.2375, 22.4477) construction
  line L279 (-79.2375, 22.4477) -> (-79.2375, 25.2375) construction
  line L280 (84, 30) -> (84, 145)
  line L281 (-84, 30) -> (-84, 145)
  line L282 (-84, 145) -> (84, 145)
  line L283 (0, -10) -> (-20, -10)
  circle A300 centre (-10, 0) radius 2.63
  circle A301 centre (10, 0) radius 2.63
  circle A302 centre (74, 60) radius 2.63
  circle A303 centre (74, 40) radius 2.63
  circle A304 centre (-74, 60) radius 2.63
  circle A305 centre (-74, 40) radius 2.63
  point P0 (0, 0)
  dimension "d0" = 5.26
  constraints: 10 end point, 6 centre point, 5 equal radius, 4 coincident, 3 horizontal, 3 point on line, 2 concentric, 2 vertical, 1 midpoint
  measures "d0" diameter of A300
ref_plane "Work Plane2" through (-78, 145, 63.1125) normal (0, 0, 1) x (1, 0, 0)
extrude "Extrusion1" add sketch "Sketch1" along normal up to surface (63.1125 mm away)
sketch "Sketch3" plane through (-84, 145, 63.1125) normal (0, 0, 1) x (1, 0, 0)
  line L0 (139.7701, -152.7549) -> (134.35, -155) projected
  line L1 (165.7549, -126.7701) -> (139.7701, -152.7549) projected
  line L2 (168, -121.35) -> (165.7549, -126.7701) projected
  line L3 (168, 0) -> (168, -121.35) projected
  line L4 (0, 0) -> (168, 0) projected
  line L5 (0, -121.35) -> (0, 0) projected
  line L6 (2.2451, -126.7701) -> (0, -121.35) projected
  line L7 (28.2299, -152.7549) -> (2.2451, -126.7701) projected
  line L8 (33.65, -155) -> (28.2299, -152.7549) projected
  line L9 (134.35, -155) -> (33.65, -155) projected
  circle A0 centre (74, -145) radius 2.63 projected
  circle A1 centre (94, -145) radius 2.63 projected
  circle A2 centre (158, -85) radius 2.63 projected
  circle A3 centre (158, -105) radius 2.63 projected
  circle A4 centre (10, -85) radius 2.63 projected
  circle A5 centre (10, -105) radius 2.63 projected
  circle A6 centre (158, -85) radius 4.5
  circle A7 centre (158, -105) radius 4.5
  circle A8 centre (94, -145) radius 4.5
  circle A9 centre (74, -145) radius 4.5
  circle A10 centre (10, -105) radius 4.5
  circle A11 centre (10, -85) radius 4.5
  point P0 (84, -145)
  dimension "d7" = 9
  constraints: 6 centre point, 6 coincident, 5 equal radius
  measures "d7" diameter of A6
extrude "Extrusion2" cut sketch "Sketch3" against normal blind 60.119 contours A6 | A7 | A8 | A9 | A10 | A11
chamfer "Chamfer2" distance 4.7625 angle 45 7 edges at (-84, 84.325, 63.1125) (-68.7625, 5.2375, 63.1125) (-53.06, -8.8775, 63.1125) (0, -10, 63.1125) (68.7625, 5.2375, 63.1125) (82.8775, 20.94, 63.1125) (84, 84.325, 63.1125)
shell "Shell1" thickness 3.5 removed faces 1 at (24.0105, 117.248, 0)
sketch "Sketch4" plane through (-84, 145, 0) normal (0, 1, 0) x (1, 0, 0)
  line L0 (164.5, -56.9003) -> (161.7878, -59.6125) projected
  line L1 (6.2122, -59.6125) -> (161.7878, -59.6125) projected
  line L2 (6.2122, -59.6125) -> (3.5, -56.9003) projected
  line L3 (3.5, 0) -> (3.5, -56.9003) projected
  line L4 (164.5, 0) -> (3.5, 0) projected
  line L5 (164.5, 0) -> (164.5, -56.9003) projected
  point P0 (84, 0)
extrude "Extrusion3" cut sketch "Sketch4" against normal blind 57.119
sketch "Sketch5" plane through (-79.2375, 145, 63.1125) normal (0, 1, 0) x (1, 0, 0)
  circle A0 centre (155.1074, 8.1301) radius 6.6301
  circle A1 centre (155.1074, 8.1301) radius 8.1301 construction
  line L0 (0, 0) -> (158.475, 0) projected
  line L1 (163.2375, 63.1125) -> (163.2375, 4.7625) projected
  line L2 (163.2375, 4.7625) -> (158.475, 0) projected
  point P0 (79.2375, 63.1125)
  dimension "d16" = 1.5
  constraints: 3 tangent, 2 centre point
  measures "d16" radial gap between concentric circles of A0 A1
extrude "Extrusion4" cut sketch "Sketch5" against normal blind 6
ref_plane "Work Plane3" through (0, 24.3462, 0) normal (-1, 0, 0) x (0, 0, 1)
mirror "Mirror1" about plane through (0, 24.3462, 0) normal (-1, 0, 0) of "Extrusion4"
sketch "Sketch6" plane through (-79.2375, 145, 63.1125) normal (0, 0, 1) x (1, 0, 0)
  circle A0 centre (79.2375, -25.4) radius 9.525
  line L0 (-4.7625, 0) -> (-4.7625, -121.35) projected
  line L1 (163.2375, -121.35) -> (163.2375, 0) projected
  line L2 (0, 0) -> (158.475, 0) projected
  point P0 (79.2375, -145)
  dimension "d19" = 19.05
  dimension "d20" = 168
  dimension "d21" = 84
  dimension "d22" = 25.4
  constraints: 1 centre point
  measures "d19" diameter of A0
  measures "d20" distance between parallel lines of L0 L1
  measures "d21" distance from line of A0.centre L1
  measures "d22" distance from line of L2 A0.centre
extrude "Extrusion5" cut sketch "Sketch6" against normal through all
fillet "Fillet1" radius 1.5875 12 edges at (80.5, 64.6637, 29.9469) (80.5, 64.6637, 1.4968) (5.3363, -6.5, 1.4968) (5.3363, -6.5, 29.9469) (-5.3363, -6.5, 29.9469) (-5.3363, -6.5, 1.4968) (14.6637, -6.5, 29.9469) (14.6637, -6.5, 1.4968) (-14.6637, -6.5, 1.4968) (-14.6637, -6.5, 29.9469) (-80.5, 64.6637, 1.4968) (-80.5, 64.6637, 29.9469)